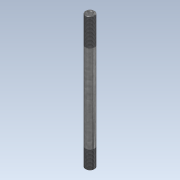
# Autodesk Inventor part: EjeManzanaD
Saved by Autodesk Inventor 2021 (Build 250183000, 183)
## iProperties
Created: 2016-06-28
Part Number: EjeManzanaD
Material: Steel
Document SubType Name: Modeling
Designer: YeseF
Density: 7.85 g/cm^3
Appearance: Steel Galvanized
Mass: 63.5599 g
Surface Area: 69.2664 cm^2
Volume: 8.09681 cm^3
Author: YeseF
Autodesk Inventor part; units mm, degrees
ref_plane "YZ Plane" through (0, 0, 0) normal (1, 0, 0) x (0, 1, 0)
ref_plane "XZ Plane" through (0, 0, 0) normal (0, 1, 0) x (-1, 0, 0)
sketch "Sketch1" plane through (0, 0, 0) normal (0, 0, 1) x (1, 0, 0)
  circle A0 centre (0, 0) radius 4.93
  circle A1 centre (0, 0) radius 2.56
  dimension "d0" = 9.86
  dimension "d1" = 5.12
  constraints: 2 centre point, 2 coincident
  measures "d0" diameter of A0
  measures "d1" diameter of A1
extrude "Extrusion1" add sketch "Sketch1" along normal blind 145.4
thread "Thread1" size "M9x1.25" class "6g" standard "ANSI Metric M Profile" length 20
ref_plane "Work Plane1" through (0, 0, 72.7) normal (0, 0, 1) x (1, 0, 0)
thread "Thread2" size "M9x1.25" class "6g" standard "ANSI Metric M Profile" length 30
chamfer "Chamfer2" distance 0.5 angle 45 4 edges at (-2.56, 0, 145.4) (-4.93, 0, 145.4) (-4.93, 0, 0) (-2.56, 0, 0)
body "Solid1"
